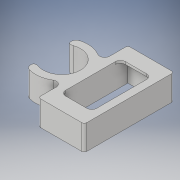
# Autodesk Inventor part: clip
Saved by Autodesk Inventor 2019 (Build 230136000, 136)
## iProperties
Created: 2020-11-09
Part Number: clip
Material: Generic
Document SubType Name: Modeling
Designer: Mike
Density: 1 g/cm^3
Appearance: Default
Author: Mike
## iProperties of the stored document clip_3DPrint.ipt
Created: 2020-11-09
Part Number: clip_3DPrint
Material: Generic
Document SubType Name: Modeling
Designer: Mike
Density: 1 g/cm^3
Appearance: Default
Author: Mike
Autodesk Inventor part; units mm, degrees
ref_plane "YZ Plane" through (0, 0, 0) normal (1, 0, 0) x (0, 1, 0)
ref_plane "XZ Plane" through (0, 0, 0) normal (0, 1, 0) x (-1, 0, 0)
ref_plane "XY Plane" through (0, 0, 0) normal (0, 0, 1) x (1, 0, 0)
sketch "Sketch1" plane through (0, 0, 0) normal (0, 1, 0) x (-1, 0, 0)
  arc A0 (3.75, 6.4952) -> (3.75, -6.4952) centre (0, 0) ccw
  arc A1 (5.25, 9.0933) -> (5.25, -9.0933) centre (0, 0) ccw
  line L0 (-11.5, 15) -> (-24, 15)
  line L1 (-24, 15) -> (-24, -15)
  line L2 (-24, -15) -> (-11.5, -15)
  line L3 (-11.5, -15) -> (-11.5, 15)
  line L4 (-8.5, 18) -> (-27, 18)
  line L5 (-27, 18) -> (-27, -18)
  line L6 (-27, -18) -> (-8.5, -18)
  line L7 (-8.5, -18) -> (-8.5, 18)
  line L8 (0, 0) -> (5.25, 9.0933)
  line L9 (0, 0) -> (10.5, 0) construction
  line L10 (5.25, 9.0933) -> (0, 0)
  line L11 (0, 0) -> (5.25, -9.0933)
  line L12 (0, 0) -> (10.5, 0) construction
  dimension "d0" = 15
  dimension "d1" = 3
  dimension "d2" = 12.5
  dimension "d3" = 30
  dimension "d4" = 3
  dimension "d5" = 3
  dimension "d6" = 3
  dimension "d7" = 3
  dimension "d8" = 15
  dimension "d9" = 11.5
  dimension "d10" = 60
  dimension "d11" = 60
  constraints: 26 end point, 7 equal length, 4 horizontal, 4 point on circle, 2 centre point, 2 coincident, 2 perpendicular, 2 point on line
  measures "d0" diameter of A0
  measures "d1" radial gap between concentric circles of A1 A0
  measures "d2" distance of L2.end L1.end
  measures "d3" distance of L1.end L0.end
  measures "d4" distance between parallel lines of L4 L0
  measures "d5" distance between parallel lines of L7 L3
  measures "d6" distance between parallel lines of L6 L2
  measures "d7" distance between parallel lines of L1 L5
  measures "d8" distance from line of point (0, 0) L0
  measures "d9" distance from line of L3 L8.start
  measures "d10" angle of L9 L8
  measures "d11" angle of L11 L12
extrude "Extrusion1" add sketch "Sketch1" along normal blind 10 contours A0 L11 A1 L7 L8 | L7 A1 | A1 L7 L6 L5 L4
fillet "Fillet1" radius 2 4 edges at (-5.25, 5, 9.0933) (-3.75, 5, 6.4952) (-5.25, 5, -9.0933) (-3.75, 5, -6.4952)
fillet "Fillet2" radius 2 2 edges at (8.5, 5, 6.1644) (8.5, 5, -6.1644)
fillet "Fillet3" radius 1 4 edges at (8.5, 5, 18) (27, 5, 18) (8.5, 5, -18) (27, 5, -18)
sketch "Sketch2" plane through (0, 10, 0) normal (0, 1, 0) x (1, 0, 0)
  line L0 (11.5, -15) -> (11.5, 15) projected
  line L1 (11.5, 15) -> (24, 15) projected
  line L2 (24, 15) -> (24, -15) projected
  line L3 (24, -15) -> (11.5, -15) projected
  arc A0 (27, 17) -> (26, 18) centre (26, 17) ccw projected
  line L4 (26, 18) -> (9.5, 18) projected
  arc A1 (9.5, 18) -> (8.5, 17) centre (9.5, 17) ccw projected
  line L5 (8.5, 17) -> (8.5, 10.6771) projected
  arc A2 (5.46, 8.9687) -> (8.5, 10.6771) centre (6.5, 10.6771) ccw projected
  arc A3 (5.46, 8.9687) -> (-2.963, 10.0733) centre (0, 0) ccw projected
  arc A4 (-2.963, 10.0733) -> (-4.1307, 7.1545) centre (-2.3986, 8.1545) ccw projected
  arc A5 (-4.1307, 7.1545) -> (-2.5443, 7.0552) centre (-3.2228, 8.9366) ccw projected
  arc A6 (-2.5443, -7.0552) -> (-2.5443, 7.0552) centre (0, 0) ccw projected
  arc A7 (-2.5443, -7.0552) -> (-4.1307, -7.1545) centre (-3.2228, -8.9366) ccw projected
  arc A8 (-4.1307, -7.1545) -> (-2.963, -10.0733) centre (-2.3986, -8.1545) ccw projected
  arc A9 (-2.963, -10.0733) -> (5.46, -8.9687) centre (0, 0) ccw projected
  arc A10 (8.5, -10.6771) -> (5.46, -8.9687) centre (6.5, -10.6771) ccw projected
  line L6 (8.5, -10.6771) -> (8.5, -17) projected
  arc A11 (8.5, -17) -> (9.5, -18) centre (9.5, -17) ccw projected
  line L7 (9.5, -18) -> (26, -18) projected
  arc A12 (26, -18) -> (27, -17) centre (26, -17) ccw projected
  line L8 (27, -17) -> (27, 17) projected
  line L9 (11.5, 15) -> (24, 15)
  line L10 (24, 15) -> (24, 12)
  line L11 (24, 12) -> (11.5, 12)
  line L12 (11.5, 12) -> (11.5, 15)
  line L13 (11.5, -15) -> (24, -15)
  line L14 (24, -15) -> (24, -12)
  line L15 (24, -12) -> (11.5, -12)
  line L16 (11.5, -12) -> (11.5, -15)
  dimension "d17" = 3
  dimension "d18" = 3
  constraints: 16 end point, 4 parallel, 2 horizontal, 2 perpendicular, 2 point on line
  measures "d17" distance of L9.end L10.end
  measures "d18" distance of L14.end L13.end
extrude "Extrusion2" add sketch "Sketch2" against normal blind 1 contours L0 L15 L2 L3 | L0 L1 L2 L11
fillet "Fillet4" radius 2 4 edges at (11.5, 9.5, -12) (24, 9.5, -12) (11.5, 9.5, 12) (24, 9.5, 12)
equation "\"d5\" = d4"
equation "\"d6\" = d4"
equation "\"d7\" = d4"
equation "\"d8\" = 0.5 * d3"
body "Solid1"
